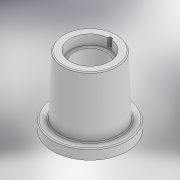
# Autodesk Inventor part: 底座
Saved by Autodesk Inventor 2020 (Build 240168000, 168)
## iProperties
Created: 2021-04-28
Part Number: 底座
Material: 常规
Document SubType Name: Modeling
Designer: Luorily
Density: 1 g/cm^3
Appearance: 默认
Author: Luorily
Autodesk Inventor part; units mm, degrees
ref_plane "YZ Plane" through (0, 0, 0) normal (1, 0, 0) x (0, 1, 0)
ref_plane "XZ Plane" through (0, 0, 0) normal (0, 1, 0) x (-1, 0, 0)
ref_plane "XY Plane" through (0, 0, 0) normal (0, 0, 1) x (1, 0, 0)
sketch "草图1" plane through (0, 0, 0) normal (0, 0, 1) x (1, 0, 0)
  line L0 (0, 0) -> (57, 0)
  line L1 (57, 0) -> (75, 0)
  line L2 (75, 0) -> (75, 20)
  line L3 (0, 0) -> (0, 140)
  line L4 (0, 140) -> (55, 140)
  line L5 (0, 140) -> (40, 140)
  line L6 (40, 140) -> (40, 120)
  line L7 (40, 120) -> (32.5, 120)
  line L8 (32.5, 120) -> (32.5, 60)
  line L9 (32.5, 60) -> (40, 60)
  line L10 (57, 0) -> (57, 3)
  line L11 (57, 3) -> (0, 3)
  line L12 (0, 3) -> (43, 3)
  line L13 (43, 3) -> (40, 60)
  line L14 (75, 20) -> (0, 20)
  line L15 (0, 20) -> (60, 20)
  line L16 (60, 20) -> (55, 140)
  dimension "d0" = 57
  dimension "d1" = 18
  dimension "d2" = 20
  dimension "d3" = 140
  dimension "d4" = 55
  dimension "d5" = 40
  dimension "d6" = 20
  dimension "d7" = 7.5
  dimension "d10" = 7.5
  dimension "d11" = 3
  dimension "d12" = 43
  dimension "d13" = 60
  constraints: 34 end point, 8 perpendicular, 6 point on line, 1 horizontal, 1 vertical
  measures "d0" distance of L0.start L0.end
  measures "d1" distance of L0.end L1.end
  measures "d2" distance of L1.end L2.end
  measures "d3" distance of L0.start L3.end
  measures "d4" distance of L3.end L4.end
  measures "d5" distance of L3.end L5.end
  measures "d6" distance of L5.end L6.end
  measures "d7" distance of L6.end L7.end
  measures "d10" distance of L8.end L9.end
  measures "d11" distance of L0.end L10.end
  measures "d12" distance of L11.end L12.end
  measures "d13" distance of L14.end L15.end
revolve "旋转1" add sketch "草图1" angle 360 about axis through (0, 0, 0) along (0, 1, 0) contours L10 L11 L13 L14 L2 L1 | L13 L9 L8 L7 L6 L4 L16 L14
fillet "圆角1" radius 2 1 edges at (-75, 20, 0)
fillet "圆角2" radius 2 1 edges at (-60, 20, 0)
fillet "圆角3" radius 2 1 edges at (-55, 140, 0)
sketch "草图2" plane through (0, 140, 0) normal (0, 1, 0) x (1, 0, 0)
  circle A0 centre (0, 0) radius 40 projected
  point P0 (0, 40)
  constraints: 1 vertical alignment, 1 other
hole "孔1" at (0, 140, -40) direction (0, -1, 0) diameter 8.376 depth 17 thread size "M10x1.5" designation "M10" class "6H" standard "GB Metric profile"
